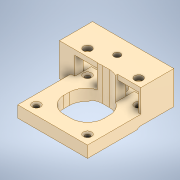
# Autodesk Inventor part: Soporte Motor Izq
Saved by Autodesk Inventor 2021 (Build 250183000, 183)
## iProperties
Created: 2023-01-27
Part Number: Soporte Motor Izq
Material: Polietileno, baja densidad
Document SubType Name: Modeling
Designer: Diego.labarca
Density: 0.894 g/cm^3
Appearance: Suave - Color hueso
Author: Diego.labarca
Autodesk Inventor part; units mm, degrees
ref_plane "YZ Plane" through (0, 0, 0) normal (1, 0, 0) x (0, 1, 0)
ref_plane "XZ Plane" through (0, 0, 0) normal (0, 1, 0) x (-1, 0, 0)
ref_plane "XY Plane" through (0, 0, 0) normal (0, 0, 1) x (1, 0, 0)
sketch "Boceto1" plane through (0, 0, 0) normal (0, 0, 1) x (1, 0, 0)
  line L0 (-28.1218, 9.9396) -> (21.1782, 9.9396)
  line L1 (21.1782, 9.9396) -> (21.1782, -10.0604)
  line L2 (21.1782, -10.0604) -> (-28.1218, -10.0604)
  line L3 (-28.1218, -10.0604) -> (-28.1218, 9.9396)
  line L4 (2.6895, 0) -> (0, 0)
  line L5 (0, 0) -> (0, 2.3867)
  dimension "d0" = 20
  dimension "d1" = 49.3
  constraints: 12 end point, 2 horizontal, 2 parallel, 2 perpendicular
  measures "d0" distance of L0.end L1.end
  measures "d1" distance of L0.start L0.end
extrude "Extrusión1" add sketch "Boceto1" along normal blind 5
sketch "Boceto2" plane through (0, 0, 5) normal (0, 0, 1) x (1, 0, 0)
  line L0 (-28.1218, 9.9396) -> (-28.1218, -10.0604) projected
  line L1 (21.1782, -10.0604) -> (21.1782, 9.9396) projected
  line L2 (-28.1218, 9.9396) -> (21.1782, 9.9396)
  line L3 (21.1782, 9.9396) -> (21.1782, 6.9396)
  line L4 (21.1782, 6.9396) -> (-28.1218, 6.9396)
  line L5 (-28.1218, 6.9396) -> (-28.1218, 9.9396)
  line L6 (21.1782, -10.0604) -> (-28.1218, -10.0604)
  line L7 (-28.1218, -10.0604) -> (-28.1218, -7.0604)
  line L8 (-28.1218, -7.0604) -> (21.1782, -7.0604)
  line L9 (21.1782, -7.0604) -> (21.1782, -10.0604)
  point P0 (0, 0)
  dimension "d4" = 3
  dimension "d5" = 3
  constraints: 16 end point, 4 parallel, 2 horizontal, 2 perpendicular, 2 point on line
  measures "d4" distance between parallel lines of L2 L4
  measures "d5" distance between parallel lines of L6 L8
extrude "Extrusión2" add sketch "Boceto2" along normal blind 15 contours L2 L1 L4 L0 | L8 L1 L6 L0
sketch "Boceto3" plane through (0, 0, 5) normal (0, 0, 1) x (1, 0, 0)
  circle A0 centre (-11.8218, 0) radius 1.75
  line L0 (-28.1218, 6.9396) -> (-28.1218, -7.0604) projected
  circle A1 centre (14.1782, -0.0604) radius 1.75
  line L1 (21.1782, -7.0604) -> (21.1782, 6.9396) projected
  point P0 (0, 0)
  dimension "d8" = 3.5
  dimension "d10" = 3.5
  dimension "d16" = 7
  dimension "d17" = 33
  constraints: 2 centre point
  measures "d8" diameter of A0
  measures "d10" diameter of A1
  measures "d16" distance from line of L1 A1.centre
  measures "d17" distance from line of A0.centre L1
extrude "Extrusión3" cut sketch "Boceto3" against normal through all
sketch "Boceto4" plane through (-28.1218, 9.9396, 0) normal (0, 1, 0) x (1, 0, 0)
  circle A0 centre (25, -10) radius 2
  line L0 (49.3, -20) -> (0, -20) projected
  line L1 (49.3, 0) -> (49.3, -20) projected
  point P0 (28.1218, 0)
  dimension "d18" = 4
  dimension "d19" = 10
  dimension "d20" = 24.3
  constraints: 1 centre point
  measures "d18" diameter of A0
  measures "d19" distance from line of A0.centre L0
  measures "d20" distance from line of L1 A0.centre
extrude "Extrusión4" cut sketch "Boceto4" against normal up to surface (20 mm away)
sketch "Boceto7" plane through (0, 0, 20) normal (0, 0, 1) x (1, 0, 0)
  line L0 (-28.1218, -10.0604) -> (21.1782, -10.0604) projected
  line L1 (21.1782, 9.9396) -> (-28.1218, 9.9396) projected
  line L2 (7.1782, -10.0604) -> (-4.8218, -10.0604)
  line L3 (-4.8218, -10.0604) -> (-4.8218, 9.9396)
  line L4 (-4.8218, 9.9396) -> (7.1782, 9.9396)
  line L5 (7.1782, 9.9396) -> (7.1782, -10.0604)
  line L6 (-28.1218, -10.0604) -> (-18.8218, -10.0604)
  line L7 (-18.8218, -10.0604) -> (-18.8218, 9.9396)
  line L8 (-18.8218, 9.9396) -> (-28.1218, 9.9396)
  line L9 (-28.1218, 9.9396) -> (-28.1218, -10.0604)
  circle A0 centre (14.1782, -0.0604) radius 1.75 projected
  circle A1 centre (-11.8218, 0) radius 1.75 projected
  point P0 (0, 0)
  point P1 (-18.8218, 9.9396)
  point P2 (-4.8218, -10.0604)
  dimension "d26" = 7
  dimension "d27" = 7
  dimension "d28" = 7
  constraints: 16 end point, 4 parallel, 4 point on line, 2 horizontal, 2 perpendicular
  measures "d26" distance from line of L5 A0.centre
  measures "d27" distance from line of A1.centre L3
  measures "d28" distance from line of A1.centre L7
extrude "Extrusión6" add sketch "Boceto7" against normal blind 5 contours L9 L1 L7 L0 | L3 L1 L5 L0
sketch "Boceto8" plane through (-28.1218, 9.9396, 0) normal (0, 1, 0) x (1, 0, 0)
  circle A0 centre (43.65, -15.65) radius 2.5
  line L0 (49.3, 0) -> (49.3, -20) projected
  line L1 (49.3, -20) -> (0, -20) projected
  circle A1 centre (12.65, -15.65) radius 2.5
  point P0 (28.1218, 0)
  dimension "d31" = 5.65
  dimension "d32" = 5
  dimension "d33" = 4.35
  dimension "d36" = 5
  dimension "d37" = 31
  constraints: 2 centre point
  measures "d31" distance from line of L0 A0.centre
  measures "d32" diameter of A0
  measures "d33" distance from line of L1 A0.centre
  measures "d36" diameter of A1
  measures "d37" distance of A0.centre A1.centre
extrude "Extrusión7" cut sketch "Boceto8" against normal up to surface (3 mm away)
sketch "Boceto9" plane through (-28.1218, 9.9396, 0) normal (0, 1, 0) x (1, 0, 0)
  circle A0 centre (43.65, -15.65) radius 2.5 projected
  circle A1 centre (12.65, -15.65) radius 2.5 projected
  circle A2 centre (43.65, -15.65) radius 1.5
  circle A3 centre (12.65, -15.65) radius 2.5 projected
  circle A4 centre (12.65, -15.65) radius 1.5
  point P0 (28.1218, 0)
  point P1 (11.3, -17.7542)
  point P2 (10.236, -15)
  point P3 (44.5029, -20)
  point P4 (42.7971, -20)
  point P5 (13.5029, -20)
  point P6 (11.7971, -20)
  dimension "d38" = 3
  dimension "d39" = 3
  constraints: 2 centre point, 2 coincident, 3 other
  measures "d38" diameter of A2
  measures "d39" diameter of A4
extrude "Extrusión8" cut sketch "Boceto9" against normal up to surface (20 mm away) contours A2 | A4
sketch "Boceto10" plane through (-28.1218, -10.0604, 0) normal (0, -1, 0) x (1, 0, 0)
  line L0 (35.3, 20) -> (49.3, 20) projected
  line L1 (49.3, 20) -> (40.3, 20)
  line L2 (40.3, 20) -> (40.3, 52.3)
  line L3 (40.3, 52.3) -> (49.3, 52.3)
  line L4 (49.3, 52.3) -> (49.3, 20)
  line L5 (49.3, 52.3) -> (7, 52.3)
  line L6 (7, 52.3) -> (7, 43.3)
  line L7 (7, 43.3) -> (49.3, 43.3)
  line L8 (49.3, 43.3) -> (49.3, 52.3)
  line L9 (0, 20) -> (49.3, 20) projected
  line L10 (7, 52.3) -> (16, 52.3)
  line L11 (16, 52.3) -> (16, 20)
  line L12 (16, 20) -> (7, 20)
  line L13 (7, 20) -> (7, 52.3)
  point P0 (28.1218, 0)
  point P1 (16, 43.3)
  point P2 (40.3, 43.3)
  dimension "d42" = 9
  dimension "d43" = 32.3
  dimension "d46" = 42.3
  dimension "d47" = 9
  dimension "d48" = 9
  constraints: 24 end point, 6 parallel, 3 horizontal, 3 perpendicular, 1 point on line
  measures "d42" distance of L2.end L3.end
  measures "d43" distance of L1.end L2.end
  measures "d46" distance of L7.end L6.end
  measures "d47" distance of L6.end L5.end
  measures "d48" distance of L11.end L12.end
extrude "Extrusión9" add sketch "Boceto10" against normal up to surface (3 mm away) contours L2 L7 L4 L0 | L9 L13 L7 L11 | L7 L11 L5 L2 | L2 L3 L4 L7 | L7 L6 L5 L11
pattern_linear "Patrón rectangular1" count 2 spacing 31 along (0, 0, 1) of "Extrusión8"
sketch "Boceto11" plane through (-28.1218, -10.0604, 0) normal (0, -1, 0) x (1, 0, 0)
  circle A0 centre (12.65, 46.65) radius 1.5 projected
  circle A1 centre (43.65, 46.65) radius 1.5 projected
  line L0 (16, 20) -> (40.3, 20) projected
  line L1 (16, 20) -> (16, 43.3) projected
  line L2 (16, 43.3) -> (40.3, 43.3) projected
  line L3 (40.3, 43.3) -> (40.3, 20) projected
  circle A2 centre (12.65, 15.65) radius 1.5 projected
  circle A3 centre (43.65, 15.65) radius 1.5 projected
  line L4 (49.3, 0) -> (49.3, 52.3) projected
  line L5 (49.3, 52.3) -> (7, 52.3) projected
  line L6 (7, 52.3) -> (7, 20) projected
  line L7 (0, 20) -> (7, 20) projected
  line L8 (0, 0) -> (0, 20) projected
  line L9 (0, 0) -> (49.3, 0) projected
  line L10 (7, 52.3) -> (7, 20) projected
  line L11 (7, 22.3) -> (49.3, 22.3)
  point P0 (28.1218, 0)
  point P1 (40.3, 22.3)
  point P2 (16, 22.3)
  dimension "d52" = 30
  constraints: 2 end point, 2 point on line, 1 perpendicular
  measures "d52" distance between parallel lines of L5 L11
extrude "Extrusión10" add sketch "Boceto11" along normal blind 1 contours L11 L6 L5 L4 L3 L2 L1
fillet "Empalme1" radius 3 2 edges at (-16.6218, -10.0604, 22.3) (16.6782, -10.0604, 22.3)
sketch "Boceto12" plane through (-28.1218, 9.9396, 0) normal (0, 1, 0) x (1, 0, 0)
  line L0 (49.3, 0) -> (49.3, -20) projected
  line L1 (49.3, -5) -> (0, -5) projected
  line L2 (49.3, -20) -> (47.8, -20)
  line L3 (47.8, -20) -> (47.8, -5)
  line L4 (47.8, -5) -> (49.3, -5)
  line L5 (49.3, -5) -> (49.3, -20)
  point P0 (28.1218, 0)
  dimension "d56" = 1.5
  constraints: 8 end point, 2 parallel, 1 horizontal, 1 perpendicular, 1 point on line
  measures "d56" distance of L3.end L4.end
extrude "Extrusión11" add sketch "Boceto12" against normal up to surface (17 mm away)
fillet "Empalme2" radius 10 4 edges at (-12.1218, -9.0604, 43.3) (-12.1218, -8.5604, 20) (12.1782, -8.5604, 20) (12.1782, -9.0604, 43.3)
sketch "Boceto13" plane through (-28.1218, -7.0604, 15) normal (0, 1, 0) x (1, 0, 0)
  line L0 (47.8, -5) -> (47.8, 10) projected
  line L1 (0, 10) -> (47.8, 10) projected
  line L2 (0, 10) -> (0, 0) projected
  line L3 (0, 0) -> (9.3, 0) projected
  line L4 (9.3, 0) -> (9.3, -5) projected
  line L5 (7, -5) -> (9.3, -5) projected
  line L6 (7, -37.3) -> (7, -5) projected
  line L7 (49.3, -37.3) -> (7, -37.3) projected
  line L8 (49.3, -5) -> (49.3, -37.3) projected
  line L9 (49.3, -5) -> (47.8, -5) projected
  circle A0 centre (12.65, -31.65) radius 1.5 projected
  circle A1 centre (43.65, -31.65) radius 1.5 projected
  circle A2 centre (12.65, -0.65) radius 1.5 projected
  circle A3 centre (43.65, -0.65) radius 1.5 projected
  line L10 (26, -28.3) -> (30.3, -28.3) projected
  arc A4 (16, -18.3) -> (26, -28.3) centre (26, -18.3) ccw projected
  line L11 (16, -15) -> (16, -18.3) projected
  arc A5 (23.3, -5.3714) -> (16, -15) centre (26, -15) ccw projected
  line L12 (23.3, -5.3714) -> (23.3, 0) projected
  line L13 (23.3, 0) -> (35.3, 0) projected
  line L14 (35.3, 0) -> (35.3, -6.3397) projected
  arc A6 (40.3, -15) -> (35.3, -6.3397) centre (30.3, -15) ccw projected
  line L15 (40.3, -18.3) -> (40.3, -15) projected
  arc A7 (30.3, -28.3) -> (40.3, -18.3) centre (30.3, -18.3) ccw projected
  line L16 (49.3, -5) -> (49.3, -37.3) projected
  line L17 (35.3, 0) -> (35.3, -6.3397) projected
  line L18 (7, -37.3) -> (7, -5) projected
  line L19 (23.3, -5.3714) -> (23.3, 0) projected
  line L20 (35.3, 0) -> (35.3, 5)
  line L21 (23.3, 0) -> (35.3, 0) projected
  line L22 (23.3, 0) -> (23.3, 5)
  line L23 (23.3, 5) -> (9.3, 5)
  line L24 (9.3, 5) -> (9.3, 0)
  line L25 (35.3, 5) -> (47.8, 5)
  line L26 (47.8, -5) -> (47.8, 10) projected
  point P0 (28.1218, 15)
  dimension "d62" = 5
  dimension "d64" = 5
  dimension "d65" = 90
  constraints: 10 end point, 2 perpendicular, 2 vertical, 1 point on line
  measures "d62" distance of L13.end L20.end
  measures "d64" distance of L12.end L22.end
  measures "d65" angle of L23 L22
extrude "Extrusión12" add sketch "Boceto13" along normal blind 3 contours L9 L8 L7 L6 L5 L4 L24 L23 L22 L12 A5 L11 A4 L10 A7 L15 A6 L14 L20 L25 L0
chamfer "Chaflán1" distance 1 angle 45 4 edges at (14.0282, -4.0604, 46.65) (-16.9718, -4.0604, 46.65) (-16.9718, -4.0604, 15.65) (14.0282, -4.0604, 15.65)
sketch "Boceto14" plane through (-28.1218, 9.9396, 0) normal (0, 1, 0) x (1, 0, 0)
  circle A0 centre (25, -10) radius 2 projected
  circle A1 centre (25, -10) radius 5
  point P0 (28.1218, 0)
  dimension "d69" = 10
  constraints: 1 centre point, 1 coincident
  measures "d69" diameter of A1
extrude "Extrusión13" add sketch "Boceto14" against normal up to surface (17 mm away)
equation "\"d10\" = d8"
equation "\"d36\" = d32"
equation "\"d39\" = d38"
